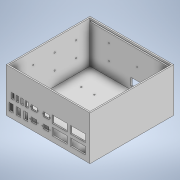
# Autodesk Inventor part: box but slightly bigger
Saved by Autodesk Inventor 2020 (Build 240168000, 168)
## iProperties
Created: 2020-01-15
Part Number: box but slightly bigger
Material: Generic
Document SubType Name: Modeling
Designer: ColinP
Density: 1 g/cm^3
Appearance: Default
Author: ColinP
Autodesk Inventor part; units mm, degrees
ref_plane "YZ Plane" through (0, 0, 0) normal (1, 0, 0) x (0, 1, 0)
ref_plane "XZ Plane" through (0, 0, 0) normal (0, 1, 0) x (-1, 0, 0)
ref_plane "XY Plane" through (0, 0, 0) normal (0, 0, 1) x (1, 0, 0)
sketch "Sketch1" plane through (0, 0, 0) normal (0, 1, 0) x (-1, 0, 0)
  line L0 (0, 0) -> (0, 127)
  line L1 (0, 127) -> (127, 127)
  line L2 (127, 127) -> (127, -127)
  line L3 (127, -127) -> (-127, -127)
  line L4 (0, 127) -> (-127, 127)
  line L5 (-127, 127) -> (-127, -127)
  dimension "d0" = 127
  dimension "d1" = 127
  dimension "d2" = 254
  dimension "d3" = 254
  dimension "d4" = 127
  constraints: 12 end point, 3 perpendicular, 1 horizontal, 1 vertical
  measures "d0" distance of L0.start L0.end
  measures "d1" distance of L0.end L1.end
  measures "d2" distance of L1.end L2.end
  measures "d3" distance of L2.end L3.end
  measures "d4" distance of L0.end L4.end
extrude "Extrusion1" add sketch "Sketch1" along normal blind 6.35
sketch "Sketch2" plane through (0, 6.35, 0) normal (0, 1, 0) x (1, 0, 0)
  line L0 (-127, -127) -> (127, -127) projected
  line L1 (-127, -127) -> (-127, -123)
  line L2 (-127, 127) -> (-127, -127) projected
  line L3 (-127, -123) -> (-123, -123)
  line L4 (-123, -123) -> (-123, 123)
  line L5 (-123, 123) -> (123, 123)
  line L6 (127, 127) -> (-127, 127) projected
  line L7 (123, 123) -> (123, -123)
  line L8 (123, -123) -> (-123, -123)
  line L9 (-127, -127) -> (127, -127)
  line L10 (127, 127) -> (127, -127)
  line L11 (-127, 127) -> (127, 127)
  line L12 (-127, 127) -> (-127, -127)
  point P0 (0, 0)
  dimension "d7" = 4
  dimension "d8" = 4
  dimension "d9" = 246
  dimension "d10" = 246
  dimension "d11" = 90
  constraints: 20 end point, 5 perpendicular, 2 collinear, 2 point on line, 1 horizontal, 1 parallel
  measures "d7" distance of L0.start L1.end
  measures "d8" distance of L1.end L3.end
  measures "d9" distance of L3.end L4.end
  measures "d10" distance of L4.end L5.end
  measures "d11" angle of L4 L5
extrude "Extrusion2" add sketch "Sketch2" along normal blind 127
sketch "Sketch3" plane through (-127, 0, 127) normal (0, 0, 1) x (1, 0, 0)
  line L0 (4, 6.35) -> (250, 6.35) projected
  line L1 (250, 6.35) -> (250, 16.35)
  line L2 (250, 6.35) -> (250, 133.35) projected
  line L3 (250, 16.35) -> (240, 16.35)
  line L4 (240, 16.35) -> (195, 16.35)
  line L5 (195, 16.35) -> (195, 38.854)
  line L6 (195, 38.854) -> (240, 38.854)
  line L7 (240, 38.854) -> (240, 16.35)
  line L8 (240, 38.854) -> (240, 48.854)
  line L9 (240, 48.854) -> (195, 48.854)
  line L10 (195, 48.854) -> (195, 71.358)
  line L11 (195, 71.358) -> (240, 71.358)
  line L12 (240, 71.358) -> (240, 48.854)
  line L13 (195, 48.854) -> (185, 48.854)
  line L14 (185, 48.854) -> (185, 71.358)
  line L15 (185, 71.358) -> (140, 71.358)
  line L16 (140, 71.358) -> (140, 48.854)
  line L17 (140, 48.854) -> (185, 48.854)
  line L18 (185, 48.854) -> (185, 38.854)
  line L19 (185, 38.854) -> (140, 38.854)
  line L20 (140, 16.35) -> (140, 38.854)
  line L21 (140, 16.35) -> (185, 16.35)
  line L22 (185, 16.35) -> (185, 38.854)
  point P0 (127, 0)
  dimension "d14" = 10
  dimension "d15" = 10
  dimension "d16" = 45
  dimension "d17" = 22.504
  dimension "d18" = 10
  dimension "d19" = 22.504
  dimension "d20" = 10
  dimension "d21" = 45
  constraints: 42 end point, 15 point on line, 12 perpendicular, 2 horizontal
  measures "d14" distance of L0.end L1.end
  measures "d15" distance of L1.end L3.end
  measures "d16" distance of L3.end L4.end
  measures "d17" distance of L4.end L5.end
  measures "d18" distance of L6.end L8.end
  measures "d19" distance of L9.end L10.end
  measures "d20" distance of L9.end L13.end
  measures "d21" distance of L14.end L15.end
sketch "Sketch4" plane through (-127, 0, 127) normal (0, 0, 1) x (1, 0, 0)
  line L0 (140, 71.358) -> (140, 48.854) projected
  line L1 (0, 0) -> (254, 0) projected
  line L2 (254, 0) -> (254, 133.35) projected
  line L3 (0, 133.35) -> (254, 133.35) projected
  line L4 (0, 0) -> (0, 133.35) projected
  line L5 (140, 16.35) -> (140, 38.854) projected
  line L6 (140, 60.106) -> (130, 60.106)
  line L7 (130, 60.106) -> (130, 66.556)
  line L8 (130, 66.556) -> (130, 60.106)
  line L9 (130, 60.106) -> (130, 53.656)
  line L10 (130, 66.556) -> (113.3, 66.556)
  line L11 (113.3, 66.556) -> (113.3, 53.656)
  line L12 (113.3, 53.656) -> (130, 53.656)
  line L13 (113.3, 66.556) -> (93.3, 66.556)
  line L14 (93.3, 66.556) -> (76.6, 66.556)
  line L15 (76.6, 66.556) -> (76.6, 53.656)
  line L16 (76.6, 53.656) -> (93.3, 53.656)
  line L17 (93.3, 53.656) -> (93.3, 66.556)
  line L18 (140, 27.602) -> (129.11, 27.602)
  line L19 (129.11, 27.602) -> (129.11, 34.052)
  line L20 (129.11, 34.052) -> (112.41, 34.052)
  line L21 (112.41, 34.052) -> (112.41, 21.152)
  line L22 (112.41, 21.152) -> (129.11, 21.152)
  line L23 (129.11, 21.152) -> (129.11, 27.602)
  line L24 (112.41, 34.052) -> (92.41, 34.052)
  line L25 (92.41, 34.052) -> (75.71, 34.052)
  line L26 (75.71, 21.152) -> (92.41, 21.152)
  line L27 (92.41, 21.152) -> (92.41, 34.052)
  line L28 (75.71, 34.052) -> (75.71, 21.152)
  point P0 (127, 0)
  dimension "d22" = 10
  dimension "d23" = 6.45
  dimension "d24" = 6.45
  dimension "d25" = 16.7
  dimension "d26" = 20
  dimension "d27" = 16.7
  dimension "d28" = 6.45
  dimension "d29" = 12.9
  dimension "d162" = 20
  dimension "d163" = 16.7
  dimension "d164" = 16.7
  constraints: 46 end point, 8 perpendicular, 6 horizontal, 4 equal length, 3 point on line, 2 midpoint, 2 vertical
  measures "d22" distance of L6.start L6.end
  measures "d23" distance of L6.end L7.end
  measures "d24" distance of L6.end L9.end
  measures "d25" distance of L7.end L10.end
  measures "d26" distance of L10.end L13.end
  measures "d27" distance of L16.end L15.end
  measures "d28" distance of L18.end L19.end
  measures "d29" distance of L20.end L21.end
  measures "d162" distance of L20.end L24.end
  measures "d163" distance of L24.end L25.end
  measures "d164" distance of L26.start L26.end
extrude "Extrusion4" cut sketch "Sketch4" against normal blind 101.6 contours L9 L12 L11 L10 L7 | L17 L16 L15 L14 | L23 L22 L21 L20 L19 | L27 L26 L28 L25
extrude "Extrusion5" cut sketch "Sketch3" against normal blind 19
sketch "Sketch6" plane through (-127, 0, 127) normal (0, 0, 1) x (1, 0, 0)
  line L0 (76.6, 53.656) -> (76.6, 66.556) projected
  line L1 (76.6, 60.106) -> (66.6, 60.106)
  line L2 (66.6, 60.106) -> (66.6, 51.756)
  line L3 (66.6, 51.756) -> (58.5, 51.756)
  line L4 (58.5, 51.756) -> (58.5, 68.456)
  line L5 (58.5, 68.456) -> (66.6, 68.456)
  line L6 (66.6, 68.456) -> (66.6, 60.106)
  line L7 (58.5, 68.456) -> (55.4, 68.456)
  line L8 (55.4, 68.456) -> (52.3, 68.456)
  line L9 (52.3, 68.456) -> (44.2, 68.456)
  line L10 (44.2, 68.456) -> (44.2, 51.756)
  line L11 (44.2, 51.756) -> (52.3, 51.756)
  line L12 (52.3, 51.756) -> (52.3, 68.456)
  line L13 (44.2, 68.456) -> (38, 68.456)
  line L14 (38, 68.456) -> (29.9, 68.456)
  line L15 (29.9, 68.456) -> (29.9, 51.756)
  line L16 (29.9, 51.756) -> (38, 51.756)
  line L17 (38, 51.756) -> (38, 68.456)
  line L18 (29.9, 68.456) -> (23.7, 68.456)
  line L19 (23.7, 68.456) -> (15.6, 68.456)
  line L20 (15.6, 68.456) -> (15.6, 51.756)
  line L21 (15.6, 51.756) -> (23.7, 51.756)
  line L22 (23.7, 51.756) -> (23.7, 68.456)
  point P0 (127, 0)
  dimension "d38" = 10
  dimension "d39" = 8.35
  dimension "d40" = 8.1
  dimension "d41" = 16.7
  dimension "d42" = 3.1
  dimension "d43" = 3.1
  dimension "d44" = 8.1
  dimension "d45" = 6.2
  dimension "d46" = 8.1
  dimension "d47" = 6.2
  dimension "d48" = 8.1
  constraints: 44 end point, 8 perpendicular, 7 horizontal, 6 parallel, 2 point on line, 1 midpoint
  measures "d38" distance of L1.start L1.end
  measures "d39" distance of L1.end L2.end
  measures "d40" distance of L2.end L3.end
  measures "d41" distance of L3.end L4.end
  measures "d42" distance of L4.end L7.end
  measures "d43" distance of L7.end L8.end
  measures "d44" distance of L11.end L10.end
  measures "d45" distance of L9.end L13.end
  measures "d46" distance of L16.end L15.end
  measures "d47" distance of L14.end L18.end
  measures "d48" distance of L21.end L20.end
sketch "Sketch7" plane through (-127, 0, 127) normal (0, 0, 1) x (1, 0, 0)
  line L0 (85.71, 27.602) -> (65.71, 27.602)
  line L1 (65.71, 27.602) -> (65.71, 38.852)
  line L2 (65.71, 27.602) -> (65.71, 16.352)
  line L3 (65.71, 16.352) -> (53.21, 16.352)
  line L4 (53.21, 16.352) -> (53.21, 38.852)
  line L5 (53.21, 38.852) -> (65.71, 38.852)
  line L6 (53.21, 27.602) -> (43.21, 27.602)
  line L7 (43.21, 27.602) -> (43.21, 38.852)
  line L8 (43.21, 38.852) -> (30.71, 38.852)
  line L9 (30.71, 38.852) -> (30.71, 16.352)
  line L10 (30.71, 16.352) -> (43.21, 16.352)
  line L11 (43.21, 27.602) -> (43.21, 16.352)
  line L12 (30.71, 38.852) -> (20.71, 38.852)
  line L13 (20.71, 38.852) -> (20.71, 16.352)
  line L14 (20.71, 16.352) -> (8.21, 16.352)
  line L15 (8.21, 16.352) -> (8.21, 38.852)
  line L16 (8.21, 38.852) -> (20.71, 38.852)
  point P0 (127, 0)
  dimension "d49" = 20
  dimension "d50" = 11.25
  dimension "d51" = 11.25
  dimension "d52" = 12.5
  dimension "d53" = 10
  dimension "d54" = 12.5
  dimension "d55" = 10
  dimension "d56" = 12.5
  constraints: 34 end point, 10 perpendicular, 9 point on line, 2 horizontal, 1 midpoint, 1 vertical
  measures "d49" distance of L0.start L0.end
  measures "d50" distance of L0.end L1.end
  measures "d51" distance of L0.end L2.end
  measures "d52" distance of L2.end L3.end
  measures "d53" distance of L6.start L6.end
  measures "d54" distance of L7.end L8.end
  measures "d55" distance of L8.end L12.end
  measures "d56" distance of L13.end L14.end
extrude "Extrusion9" cut sketch "Sketch6" against normal blind 19
extrude "Extrusion11" cut sketch "Sketch7" against normal blind 10
sketch "Sketch12" plane through (0, 0, 0) normal (0, 1, 0) x (1, 0, 0)
  line L0 (-123, -123) -> (123, -123) projected
  line L1 (89.6088, -123) -> (89.6088, 4)
  line L2 (89.6088, -123) -> (216.6088, -123) construction
  line L3 (89.6088, 4) -> (89.6088, 54.8)
  line L4 (89.6088, 54.8) -> (49.6088, 54.8)
  circle A0 centre (89.6088, 54.8) radius 1.75
  circle A1 centre (49.6088, 54.8) radius 1.75
  line L5 (34.61, -135.8133) -> (161.61, -135.8133) construction
  line L6 (-61.29, -127) -> (-61.29, -123) projected
  line L7 (-61.29, -123) -> (65.71, -123) construction
  line L8 (-127, -127) -> (127, -127) projected
  line L9 (0, -127) -> (-61.5, -127)
  line L10 (-61.5, -127) -> (-61.5, -25.4)
  line L11 (-61.5, -25.4) -> (-81.5, -25.4)
  line L12 (-81.5, -25.4) -> (-41.5, -25.4)
  line L13 (-41.5, -25.4) -> (-41.5, 54.8)
  line L14 (-41.5, 54.8) -> (-81.5, 54.8)
  circle A2 centre (-41.5, -25.4) radius 1.75
  circle A3 centre (-81.5, -25.4) radius 1.75
  circle A4 centre (-81.5, 54.8) radius 1.75
  circle A5 centre (-41.5, 54.8) radius 1.75
  dimension "d84" = 127
  dimension "d85" = 90
  dimension "d86" = 50.8
  dimension "d87" = 40
  dimension "d88" = 3.5
  dimension "d89" = 3.5
  dimension "d97" = 61.5
  dimension "d98" = 101.6
  dimension "d99" = 20
  dimension "d100" = 40
  dimension "d101" = 40
  dimension "d102" = 3.5
  dimension "d103" = 3.5
  dimension "d104" = 3.5
  dimension "d105" = 3.5
  constraints: 24 end point, 6 centre point, 6 coincident, 6 perpendicular, 4 point on line, 3 horizontal, 1 midpoint, 1 vertical
  measures "d84" distance of L1.start L1.end
  measures "d85" angle of L2 L1
  measures "d86" distance of L1.end L3.end
  measures "d87" distance of L3.end L4.end
  measures "d88" diameter of A0
  measures "d89" diameter of A1
  measures "d97" distance of L9.start L9.end
  measures "d98" distance of L9.end L10.end
  measures "d99" distance of L10.end L11.end
  measures "d100" distance of L11.end L12.end
  measures "d101" distance of L13.end L14.end
  measures "d102" diameter of A2
  measures "d103" diameter of A3
  measures "d104" diameter of A4
  measures "d105" diameter of A5
sketch "Sketch13" plane through (-123, 6.35, 123) normal (1, 0, 0) x (0, 0, -1)
  line L0 (246, 127) -> (236, 127)
  line L1 (0, 127) -> (246, 127) projected
  line L2 (236, 127) -> (226, 127)
  line L3 (226, 127) -> (226, 94.3)
  line L4 (226, 94.3) -> (181, 94.3)
  line L5 (181, 94.3) -> (181, 37.3)
  line L6 (181, 37.3) -> (226, 37.3)
  line L7 (226, 37.3) -> (226, 94.3)
  line L8 (181, 94.3) -> (161, 94.3)
  line L9 (161, 94.3) -> (161, 37.3)
  line L10 (161, 37.3) -> (116, 37.3)
  line L11 (116, 37.3) -> (116, 94.3)
  line L12 (116, 94.3) -> (161, 94.3)
  line L13 (116, 94.3) -> (96, 94.3)
  line L14 (116, 94.3) -> (136, 94.3) construction
  line L15 (96, 94.3) -> (96, 37.3)
  line L16 (96, 37.3) -> (51, 37.3)
  line L17 (51, 37.3) -> (51, 94.3)
  line L18 (51, 94.3) -> (96, 94.3)
  line L19 (73.5, 94.3) -> (73.5, 89.3)
  line L20 (73.5, 37.3) -> (73.5, 42.3)
  line L21 (138.5, 94.3) -> (138.5, 89.3)
  line L22 (138.5, 89.3) -> (138.5, 42.3)
  line L23 (203.5, 94.3) -> (203.5, 89.3)
  line L24 (203.5, 89.3) -> (203.5, 42.3)
  circle A0 centre (73.5, 42.3) radius 2
  circle A1 centre (73.5, 89.3) radius 2
  circle A2 centre (138.5, 89.3) radius 2
  circle A3 centre (138.5, 42.3) radius 2
  circle A4 centre (203.5, 42.3) radius 2
  circle A5 centre (203.5, 89.3) radius 2
  line L25 (51, 94.3) -> (31, 94.3)
  line L26 (51, 94.3) -> (71, 94.3) construction
  point P0 (123, -6.35)
  dimension "d108" = 10
  dimension "d109" = 10
  dimension "d110" = 32.7
  dimension "d111" = 90
  dimension "d112" = 45
  dimension "d113" = 57
  dimension "d114" = 20
  dimension "d115" = 45
  dimension "d116" = 20
  dimension "d117" = 180
  dimension "d118" = 57
  dimension "d119" = 45
  dimension "d120" = 5
  dimension "d121" = 5
  dimension "d122" = 5
  dimension "d123" = 4
  dimension "d124" = 4
  dimension "d125" = 4
  dimension "d126" = 4
  dimension "d127" = 4
  dimension "d128" = 4
  dimension "d151" = 20
  dimension "d152" = 180
  constraints: 52 end point, 11 perpendicular, 9 point on line, 6 centre point, 6 coincident, 5 horizontal, 5 vertical, 4 midpoint, 2 collinear
  measures "d108" distance of L0.start L0.end
  measures "d109" distance of L0.end L2.end
  measures "d110" distance of L2.end L3.end
  measures "d111" angle of L3 L2
  measures "d112" distance of L3.end L4.end
  measures "d113" distance of L4.end L5.end
  measures "d114" distance of L4.end L8.end
  measures "d115" distance of L9.end L10.end
  measures "d116" distance of L11.end L13.end
  measures "d117" angle of L13 L14
  measures "d118" distance of L13.end L15.end
  measures "d119" distance of L15.end L16.end
  measures "d120" distance of L19.start L19.end
  measures "d121" distance of L20.start L20.end
  measures "d122" distance of L21.start L21.end
  measures "d123" diameter of A0
  measures "d124" diameter of A1
  measures "d125" diameter of A2
  measures "d126" diameter of A3
  measures "d127" diameter of A4
  measures "d128" diameter of A5
  measures "d151" distance of L17.end L25.end
  measures "d152" angle of L25 L26
sketch "Sketch17" plane through (-127, 0, 127) normal (0, 0, 1) x (1, 0, 0)
  line L0 (93.3, 53.656) -> (93.3, 66.556) projected
  line L1 (93.3, 60.106) -> (96.3, 60.106)
  line L2 (96.3, 60.106) -> (100.3, 60.106)
  circle A0 centre (96.3, 60.106) radius 1.5
  line L3 (76.6, 53.656) -> (76.6, 66.556) projected
  line L4 (76.6, 60.106) -> (73.6, 60.106)
  line L5 (75.71, 21.152) -> (75.71, 34.052) projected
  line L6 (75.71, 27.602) -> (72.71, 27.602)
  line L7 (92.41, 34.052) -> (92.41, 21.152) projected
  line L8 (92.41, 27.602) -> (95.41, 27.602)
  line L9 (113.3, 53.656) -> (113.3, 66.556) projected
  line L10 (113.3, 60.106) -> (110.3, 60.106)
  line L11 (112.41, 21.152) -> (112.41, 34.052) projected
  line L12 (112.41, 27.602) -> (109.41, 27.602)
  line L13 (129.11, 34.052) -> (129.11, 21.152) projected
  line L14 (129.11, 27.602) -> (132.11, 27.602)
  line L15 (130, 66.556) -> (130, 53.656) projected
  line L16 (130, 60.106) -> (133, 60.106)
  circle A1 centre (110.3, 60.106) radius 1.5
  circle A2 centre (133, 60.106) radius 1.5
  circle A3 centre (132.11, 27.602) radius 1.5
  circle A4 centre (95.41, 27.602) radius 1.5
  circle A5 centre (109.41, 27.602) radius 1.5
  circle A6 centre (72.71, 27.602) radius 1.5
  circle A7 centre (73.6, 60.106) radius 1.5
  point P0 (127, 0)
  dimension "d147" = 3
  dimension "d148" = 4
  dimension "d150" = 3
  dimension "d165" = 3
  dimension "d166" = 3
  dimension "d167" = 3
  dimension "d168" = 3
  dimension "d169" = 3
  dimension "d170" = 3
  dimension "d171" = 3
  dimension "d172" = 3
  dimension "d173" = 3
  dimension "d174" = 3
  dimension "d175" = 3
  dimension "d176" = 3
  dimension "d177" = 3
  dimension "d178" = 3
  constraints: 18 end point, 8 centre point, 8 coincident, 8 horizontal, 8 midpoint, 1 point on line
  measures "d147" distance of L1.start L1.end
  measures "d148" distance of L1.end L2.end
  measures "d150" diameter of A0
  measures "d165" distance of L4.start L4.end
  measures "d166" distance of L6.start L6.end
  measures "d167" distance of L8.start L8.end
  measures "d168" distance of L10.start L10.end
  measures "d169" distance of L12.start L12.end
  measures "d170" distance of L14.start L14.end
  measures "d171" distance of L16.start L16.end
  measures "d172" diameter of A1
  measures "d173" diameter of A2
  measures "d174" diameter of A3
  measures "d175" diameter of A4
  measures "d176" diameter of A5
  measures "d177" diameter of A6
  measures "d178" diameter of A7
sketch "Sketch18" plane through (-123, 6.35, -123) normal (0, 0, 1) x (1, 0, 0)
  line L0 (0, 127) -> (35.4, 127)
  line L1 (0, 127) -> (246, 127) projected
  line L2 (35.4, 127) -> (35.4, 94.3)
  line L3 (35.4, 94.3) -> (80.4, 94.3)
  line L4 (80.4, 94.3) -> (80.4, 37.3)
  line L5 (80.4, 37.3) -> (35.4, 37.3)
  line L6 (35.4, 37.3) -> (35.4, 94.3)
  line L7 (57.9, 94.3) -> (57.9, 89.3)
  line L8 (57.9, 89.3) -> (57.9, 42.3)
  circle A0 centre (57.9, 89.3) radius 2
  circle A1 centre (57.9, 42.3) radius 2
  point P0 (123, -6.35)
  dimension "d153" = 35.4
  dimension "d154" = 32.7
  dimension "d155" = 90
  dimension "d156" = 45
  dimension "d157" = 57
  dimension "d158" = 5
  dimension "d159" = 47
  dimension "d160" = 4
  dimension "d161" = 4
  constraints: 16 end point, 4 perpendicular, 3 point on line, 2 centre point, 2 coincident, 1 collinear, 1 midpoint, 1 vertical
  measures "d153" distance of L0.start L0.end
  measures "d154" distance of L0.end L2.end
  measures "d155" angle of L0 L2
  measures "d156" distance of L2.end L3.end
  measures "d157" distance of L3.end L4.end
  measures "d158" distance of L7.start L7.end
  measures "d159" distance of L7.end L8.end
  measures "d160" diameter of A0
  measures "d161" diameter of A1
extrude "Extrusion18" cut sketch "Sketch17" against normal blind 10
sketch "Sketch19" plane through (127, 0, -127) normal (0, 0, -1) x (-1, 0, 0)
  line L0 (4, 6.35) -> (4, 133.35) projected
  line L1 (4, 6.35) -> (64, 6.35)
  line L2 (4, 6.35) -> (250, 6.35) projected
  line L3 (64, 6.35) -> (64, 16.35)
  line L4 (64, 16.35) -> (125.6, 16.35)
  line L5 (14, 16.35) -> (59, 16.35) projected
  line L6 (125.6, 16.35) -> (125.6, 39.35)
  line L7 (125.6, 39.35) -> (64, 39.35)
  line L8 (59, 38.854) -> (14, 38.854) projected
  line L9 (64, 39.35) -> (64, 16.35)
  point P0 (127, 0)
  dimension "d204" = 60
  dimension "d205" = 10
  dimension "d206" = 61.6
  dimension "d207" = 23
  dimension "d208" = 61.6
  dimension "d209" = 90
  constraints: 12 end point, 2 perpendicular, 1 collinear, 1 parallel, 1 point on line
  measures "d204" distance of L0.start L1.end
  measures "d205" distance of L1.end L3.end
  measures "d206" distance of L3.end L4.end
  measures "d207" distance of L4.end L6.end
  measures "d208" distance of L6.end L7.end
  measures "d209" angle of L7 L6
extrude "Extrusion21" cut sketch "Sketch19" against normal blind 5
sketch "Sketch20" plane through (127, 0, -127) normal (0, 0, -1) x (-1, 0, 0)
  line L0 (44.89, 52.655) -> (106.49, 52.655)
  line L1 (44.89, 52.655) -> (106.49, 52.655) construction
  line L2 (106.49, 52.655) -> (106.49, 75.655)
  circle A0 centre (44.89, 52.655) radius 1.75
  circle A1 centre (106.49, 75.655) radius 1.75
  line L3 (61, 43.854) -> (4, 43.854) projected
  line L4 (64, 39.35) -> (125.6, 39.35) projected
  point P0 (127, 0)
  dimension "d190" = 61.6
  dimension "d191" = 0
  dimension "d192" = 23
  dimension "d193" = 90
  dimension "d194" = 3.5
  dimension "d195" = 3.5
  constraints: 6 end point, 2 centre point, 2 coincident, 1 collinear, 1 horizontal
  measures "d190" distance of L0.start L0.end
  measures "d191" distance between parallel lines of L0 L1
  measures "d192" distance of L0.end L2.end
  measures "d193" angle of L2 L0
  measures "d194" diameter of A0
  measures "d195" diameter of A1
extrude "Extrusion20" cut sketch "Sketch20" against normal blind 127
sketch "Sketch21" plane through (127, 0, -127) normal (0, 0, -1) x (-1, 0, 0)
  line L0 (0, 0) -> (0, 133.35) projected
  line L1 (0, 133.35) -> (4.2, 133.35)
  line L2 (254, 133.35) -> (0, 133.35) projected
  line L3 (250, 133.35) -> (4, 133.35) projected
  line L4 (4, 133.35) -> (4, 128.35)
  line L5 (4, 133.35) -> (9, 133.35) construction
  line L6 (254, 0) -> (254, 133.35) projected
  line L7 (254, 133.35) -> (249.8, 133.35)
  line L8 (249.8, 133.35) -> (249.8, 128.35)
  line L9 (250, 6.35) -> (250, 133.35) projected
  line L10 (249.8, 128.35) -> (4, 128.35)
  line L11 (4, 128.35) -> (4, 123.35)
  line L12 (4, 6.35) -> (4, 133.35) projected
  line L13 (4, 123.35) -> (249.8, 123.35)
  line L14 (249.8, 123.35) -> (249.8, 128.35)
  line L15 (249.8, 123.35) -> (249.8, 128.35)
  point P0 (127, 0)
  dimension "d212" = 4.2
  dimension "d213" = 5
  dimension "d214" = 90
  dimension "d215" = 4.2
  dimension "d216" = 5
  dimension "d217" = 90
  dimension "d218" = 5
  constraints: 20 end point, 4 point on line, 3 perpendicular, 1 collinear, 1 horizontal, 1 parallel, 1 vertical
  measures "d212" distance of L0.end L1.end
  measures "d213" distance of L3.end L4.end
  measures "d214" angle of L4 L5
  measures "d215" distance of L2.start L7.end
  measures "d216" distance of L7.end L8.end
  measures "d217" angle of L8 L7
  measures "d218" distance of L4.end L11.end
extrude "Extrusion22" cut sketch "Sketch21" against normal blind 5 contours L10 L14 L13 L11
extrude "Extrusion23" cut sketch "Sketch18" against normal blind 5 contours A1 | A0 L8 L7 | L7 L8 A0
extrude "Extrusion24" cut sketch "Sketch13" against normal blind 5 contours A4 | A5 L24 L23 | L23 L24 A5 | A1 | A0 | A3 | A2 L22 L21 | L21 L22 A2
hole "Hole1" at (89.6088, 0, -54.8) at (49.6088, 0, -54.8) at (-41.5, 0, -54.8) at (-81.5, 0, -54.8) at (-41.5, 0, 25.4) at (-81.5, 0, 25.4) direction (0, 1, 0) diameter 4 end through all counterbore diameter 6 counterbore depth 3
body "Solid1"
